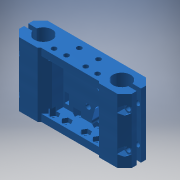
# Autodesk Inventor part: ChimeraXCarriageBushings
Saved by Autodesk Inventor 2016 (Build 200138000, 138)
## iProperties
Category: Print
Created: 2015-03-10
Part Number: ChimeraXCarriageBushings
Material: ABS Plastic
Document SubType Name: Modeling
Designer: Jack
Density: 1.06 g/cm^3
Appearance: Cyan
Mass: 40.4192 g
Surface Area: 204.208 cm^2
Volume: 38.1313 cm^3
Author: Jack
Title: Chimera X Carriage V6
Autodesk Inventor part; units mm, degrees
ref_plane "YZ Plane" through (0, 0, 0) normal (1, 0, 0) x (0, 1, 0)
ref_plane "XZ Plane" through (0, 0, 0) normal (0, 1, 0) x (-1, 0, 0)
sketch "Sketch1" plane through (0, 0, 0) normal (0, 0, 1) x (1, 0, 0)
  arc A0 (-6.0673, -1.5) -> (-6.0673, 1.5) centre (0, 0) ccw
  arc A1 (61.0673, 1.5) -> (61.0673, -1.5) centre (55, 0) ccw
  line L0 (-6.0673, -1.5) -> (-12, -1.5)
  line L1 (-12, -1.5) -> (-12, -10)
  line L2 (-12, -10) -> (11, -10)
  line L3 (11, -10) -> (11, 3)
  line L4 (11, 3) -> (44, 3)
  line L5 (44, 3) -> (44, -10)
  line L6 (44, -10) -> (67, -10)
  line L7 (67, -10) -> (67, -1.5)
  line L8 (67, -1.5) -> (61.0673, -1.5)
  line L9 (61.0673, 1.5) -> (67, 1.5)
  line L10 (67, 1.5) -> (67, 10)
  line L11 (67, 10) -> (44, 10)
  line L12 (44, 10) -> (44, 10)
  line L13 (44, 10) -> (11, 10)
  line L14 (11, 10) -> (11, 10)
  line L15 (11, 10) -> (-12, 10)
  line L16 (-12, 10) -> (-12, 1.5)
  line L17 (-12, 1.5) -> (-6.0673, 1.5)
  dimension "d0" = 12.5
  dimension "d1" = 55
  dimension "d2" = 1.5
  dimension "d4" = 10
  dimension "d5" = 11
  dimension "d6" = 10
  dimension "d8" = 13
  dimension "d9" = 7
  dimension "d147" = 12
  constraints: 36 end point, 12 perpendicular, 6 point on line, 4 equal length, 4 point on circle, 4 vertical alignment, 2 centre point, 2 horizontal alignment, 1 coincident, 1 equal radius, 1 horizontal, 1 parallel, 1 vertical
  measures "d0" diameter of A0
  measures "d1" distance of A1.centre point (0, 0)
  measures "d2" distance from line of point (0, 0) L0
  measures "d4" distance from line of L15 point (0, 0)
  measures "d5" distance from line of L14 point (0, 0)
  measures "d6" distance from line of L2 point (0, 0)
  measures "d8" distance of L2.end L3.end
  measures "d9" distance between parallel lines of L4 L13
  measures "d147" distance from line of point (0, 0) L16
extrude "Extrusion1" add sketch "Sketch1" along normal blind 45
chamfer "Chamfer1" distance 5 angle 45 6 edges at (-12, 10, 22.5) (-12, -10, 22.5) (67, -10, 22.5) (67, 10, 22.5) (44, -10, 22.5) (11, -10, 22.5)
sketch "Sketch2" plane through (-7, 10, 0) normal (0, 1, 0) x (1, 0, 0)
  line L0 (69, 0) -> (69, -45) projected
  line L1 (0, -45) -> (0, 0) projected
  line L2 (74, -45) -> (74, 0) projected
  line L3 (-5, 0) -> (-5, -45) projected
  line L4 (74, 0) -> (69, 0) projected
  line L5 (69, -45) -> (74, -45) projected
  point P0 (7, 0)
  point P1 (-2.5, -10)
  point P2 (-2.5, -35)
  point P3 (71.5, -10)
  point P4 (71.5, -35)
  dimension "d18" = 2.5
  dimension "d19" = 2.5
  dimension "d20" = 10
  dimension "d21" = 10
  constraints: 2 horizontal alignment, 2 vertical alignment
  measures "d18" distance from line of L1 point (-2.5, -10)
  measures "d19" distance from line of L0 point (71.5, -10)
  measures "d20" distance from line of L4 point (71.5, -10)
  measures "d21" distance from line of L5 point (71.5, -35)
hole "Hole1" at (-9.5, 10, 10) at (-9.5, 10, 35) at (64.5, 10, 10) at (64.5, 10, 35) direction (0, -1, 0) diameter 3.5 end through all counterbore diameter 7.3 counterbore depth 5
sketch "Sketch3" plane through (49, -10, 0) normal (0, -1, 0) x (1, 0, 0)
  circle A0 centre (15.5, 10) radius 1.75 projected
  circle A1 centre (15.5, 35) radius 1.75 projected
  circle A2 centre (-58.5, 35) radius 1.75 projected
  circle A3 centre (-58.5, 10) radius 1.75 projected
  line L0 (15.5, 13.1754) -> (18.25, 11.5877)
  line L1 (18.25, 11.5877) -> (18.25, 8.4123)
  line L2 (18.25, 8.4123) -> (15.5, 6.8246)
  line L3 (15.5, 6.8246) -> (12.75, 8.4123)
  line L4 (12.75, 8.4123) -> (12.75, 11.5877)
  line L5 (12.75, 11.5877) -> (15.5, 13.1754)
  line L6 (15.5, 31.8246) -> (12.75, 33.4123)
  line L7 (12.75, 33.4123) -> (12.75, 36.5877)
  line L8 (12.75, 36.5877) -> (15.5, 38.1754)
  line L9 (15.5, 38.1754) -> (18.25, 36.5877)
  line L10 (18.25, 36.5877) -> (18.25, 33.4123)
  line L11 (18.25, 33.4123) -> (15.5, 31.8246)
  circle A4 centre (-58.5, 10) radius 1.75 projected
  line L12 (-58.5, 6.8246) -> (-61.25, 8.4123)
  line L13 (-61.25, 8.4123) -> (-61.25, 11.5877)
  line L14 (-61.25, 11.5877) -> (-58.5, 13.1754)
  line L15 (-58.5, 13.1754) -> (-55.75, 11.5877)
  line L16 (-55.75, 11.5877) -> (-55.75, 8.4123)
  line L17 (-55.75, 8.4123) -> (-58.5, 6.8246)
  line L18 (-58.5, 38.1754) -> (-55.75, 36.5877)
  line L19 (-55.75, 36.5877) -> (-55.75, 33.4123)
  line L20 (-55.75, 33.4123) -> (-58.5, 31.8246)
  line L21 (-58.5, 31.8246) -> (-61.25, 33.4123)
  line L22 (-61.25, 33.4123) -> (-61.25, 36.5877)
  line L23 (-61.25, 36.5877) -> (-58.5, 38.1754)
  point P0 (-49, 0)
  point P1 (-58.5, 10)
  dimension "d29" = 5.5
  constraints: 48 end point, 4 coincident, 4 vertical, 3 parallel, 52 other
  measures "d29" distance between parallel lines of L4 L1
extrude "Extrusion2" cut sketch "Sketch3" against normal blind 5
sketch "Sketch5" plane through (-7, 10, 0) normal (0, 1, 0) x (1, 0, 0)
  line L0 (0, 0) -> (69, 0) projected
  line L1 (51, 0) -> (51, -45) projected
  point P0 (7, 0)
  point P1 (47.5, -22.5)
  point P2 (35.5, -31)
  point P3 (35.5, -14)
  dimension "d44" = 17
  dimension "d45" = 12
  dimension "d46" = 3.5
  dimension "d47" = 22.5
  dimension "d48" = 8.5
  constraints: 1 vertical alignment
  measures "d44" distance of point (35.5, -31) point (35.5, -14)
  measures "d45" horizontal distance of point (35.5, -14) point (47.5, -22.5)
  measures "d46" distance from line of L1 point (47.5, -22.5)
  measures "d47" distance from line of L0 point (47.5, -22.5)
  measures "d48" vertical distance of point (47.5, -22.5) point (35.5, -31)
hole "Hole3" at (40.5, 10, 22.5) at (28.5, 10, 31) at (28.5, 10, 14) direction (0, -1, 0) diameter 3.5 end through all counterbore diameter 7.3 counterbore depth 3.5
sketch "Sketch6" plane through (-7, 10, 0) normal (0, 1, 0) x (1, 0, 0)
  circle A0 centre (47.5, -22.5) radius 3.65 projected
  arc A1 (50.9105, -7.1631) -> (48.5, -4) centre (48.5, -6.5) ccw
  arc A2 (48.5, -41) -> (50.9105, -37.8369) centre (48.5, -38.5) ccw
  arc A3 (48.8388, -30.3064) -> (40.1612, -30.3064) centre (44.5, -31.5) ccw
  arc A4 (40.1612, -14.6936) -> (48.8388, -14.6936) centre (44.5, -13.5) ccw
  arc A5 (40.5, -4) -> (38.0895, -7.1631) centre (40.5, -6.5) ccw
  arc A6 (38.0895, -37.8369) -> (40.5, -41) centre (40.5, -38.5) ccw
  line L0 (40.5, -4) -> (48.5, -4)
  line L1 (50.9105, -7.1631) -> (48.8388, -14.6936)
  line L2 (38.0895, -7.1631) -> (40.1612, -14.6936)
  line L3 (48.8388, -30.3064) -> (50.9105, -37.8369)
  line L4 (40.1612, -30.3064) -> (38.0895, -37.8369)
  line L5 (40.5, -41) -> (48.5, -41)
  point P0 (7, 0)
  dimension "d136" = 9
  dimension "d138" = 4
  dimension "d139" = 9
  dimension "d140" = 9
  dimension "d141" = 18
  dimension "d142" = 3
  dimension "d143" = 7
  dimension "d144" = 7
  dimension "d145" = 5
  dimension "d146" = 4
  constraints: 12 end point, 12 point on circle, 12 tangent, 6 centre point, 3 equal radius, 3 vertical alignment, 2 horizontal alignment, 1 horizontal
  measures "d136" diameter of A3
  measures "d138" horizontal distance of A2.centre A3.centre
  measures "d139" vertical distance of A0.centre A3.centre
  measures "d140" diameter of A4
  measures "d141" distance of A3.centre A4.centre
  measures "d142" horizontal distance of A0.centre A4.centre
  measures "d143" vertical distance of A2.centre A3.centre
  measures "d144" vertical distance of A4.centre A1.centre
  measures "d145" diameter of A1
  measures "d146" horizontal distance of A4.centre A5.centre
extrude "Extrusion3" cut sketch "Sketch6" against normal up to surface (7 mm away) contours L1 A4 L2 A5 L0 A1 | L5 A6 L4 A3 L3 A2
sketch "Sketch7" plane through (0, 0, 45) normal (0, 0, 1) x (1, 0, 0)
  line L0 (11, -5) -> (6, -10) projected
  line L1 (11, -5) -> (11, 3) projected
  line L2 (11, 3) -> (44, 3) projected
  line L3 (44, 3) -> (44, -5) projected
  arc A0 (61.0673, 1.5) -> (61.0673, -1.5) centre (55, 0) ccw projected
  line L4 (7.3, -8.7) -> (47.7, -8.7)
  line L5 (44, -5) -> (49, -10) projected
  dimension "d66" = 8.7
  constraints: 2 end point, 2 point on line, 1 horizontal
  measures "d66" distance from line of A0.centre L4
extrude "Extrusion4" add sketch "Sketch7" against normal blind 5
sketch "Sketch8" plane through (0, 0, 0) normal (0, 0, -1) x (-1, 0, 0)
  line L0 (-11, -5) -> (-7.3, -8.7) projected
  line L1 (-11, 3) -> (-11, -5) projected
  line L2 (-31.5, 3) -> (-11, 3) projected
  line L3 (-44, -5) -> (-44, 3) projected
  line L4 (-47.7, -8.7) -> (-44, -5) projected
  line L5 (-47.7, -8.7) -> (-7.3, -8.7) projected
  line L6 (-31.5, 3) -> (-43.5, 3) projected
  line L7 (-44, 3) -> (-43.5, 3) projected
extrude "Extrusion5" add sketch "Sketch8" against normal blind 5
sketch "Sketch9" plane through (0, 0, 0) normal (0, 0, -1) x (-1, 0, 0)
  arc A0 (6.0673, 1.5) -> (6.0673, -1.5) centre (0, 0) ccw projected
  line L0 (12, 1.5) -> (12, 5) projected
  circle A1 centre (-34.25, 4.45) radius 1.75
  circle A2 centre (-34.25, -4.45) radius 1.75
  circle A3 centre (-20.75, 4.45) radius 1.75
  circle A4 centre (-20.75, -4.45) radius 1.75
  dimension "d71" = 3.5
  dimension "d72" = 13.5
  dimension "d73" = 8.9
  dimension "d74" = 4.45
  dimension "d76" = 32.75
  constraints: 4 centre point, 3 equal radius, 2 horizontal alignment, 2 vertical alignment
  measures "d71" diameter of A1
  measures "d72" distance of A3.centre A1.centre
  measures "d73" distance of A3.centre A4.centre
  measures "d74" vertical distance of A0.centre A3.centre
  measures "d76" distance from line of L0 A3.centre
extrude "Extrusion6" cut sketch "Sketch9" against normal up to surface (5 mm away)
sketch "Sketch10" plane through (0, 0, 45) normal (0, 0, 1) x (1, 0, 0)
  circle A0 centre (34.25, -4.45) radius 1.75 projected
  circle A1 centre (20.75, -4.45) radius 1.75 projected
  arc A2 (19.7702, 3) -> (21.7298, 3) centre (20.75, 4.45) ccw projected
  arc A3 (33.2702, 3) -> (35.2298, 3) centre (34.25, 4.45) ccw projected
  circle A4 centre (20.75, 4.45) radius 1.75 projected
  circle A5 centre (34.25, 4.45) radius 1.75 projected
extrude "Extrusion7" cut sketch "Sketch10" against normal up to surface (5 mm away)
sketch "Sketch11" plane through (0, 0, 40) normal (0, 0, -1) x (-1, 0, 0)
  arc A0 (-21.7298, 3) -> (-19.7702, 3) centre (-20.75, 4.45) ccw projected
  arc A1 (-35.2298, 3) -> (-33.2702, 3) centre (-34.25, 4.45) ccw projected
  circle A2 centre (-20.75, -4.45) radius 1.75 projected
  circle A3 centre (-34.25, -4.45) radius 1.75 projected
  line L0 (-31.5, 6.0377) -> (-31.5, 2.8623)
  line L1 (-31.5, 2.8623) -> (-34.25, 1.2746)
  line L2 (-34.25, 1.2746) -> (-37, 2.8623)
  line L3 (-37, 2.8623) -> (-37, 6.0377)
  line L4 (-37, 6.0377) -> (-34.25, 7.6254)
  line L5 (-34.25, 7.6254) -> (-31.5, 6.0377)
  line L6 (-31.0746, -4.45) -> (-32.6623, -7.2)
  line L7 (-32.6623, -7.2) -> (-35.8377, -7.2)
  line L8 (-35.8377, -7.2) -> (-37.4254, -4.45)
  line L9 (-37.4254, -4.45) -> (-35.8377, -1.7)
  line L10 (-35.8377, -1.7) -> (-32.6623, -1.7)
  line L11 (-32.6623, -1.7) -> (-31.0746, -4.45)
  line L12 (-23.9254, -4.45) -> (-22.3377, -1.7)
  line L13 (-22.3377, -1.7) -> (-19.1623, -1.7)
  line L14 (-19.1623, -1.7) -> (-17.5746, -4.45)
  line L15 (-17.5746, -4.45) -> (-19.1623, -7.2)
  line L16 (-19.1623, -7.2) -> (-22.3377, -7.2)
  line L17 (-22.3377, -7.2) -> (-23.9254, -4.45)
  line L18 (-23.5, 6.0377) -> (-20.75, 7.6254)
  line L19 (-20.75, 7.6254) -> (-18, 6.0377)
  line L20 (-18, 6.0377) -> (-18, 2.8623)
  line L21 (-18, 2.8623) -> (-20.75, 1.2746)
  line L22 (-20.75, 1.2746) -> (-23.5, 2.8623)
  line L23 (-23.5, 2.8623) -> (-23.5, 6.0377)
  point P0 (0, 0)
  dimension "d81" = 5.5
  constraints: 48 end point, 4 coincident, 3 equal length, 2 horizontal, 2 vertical, 52 other
  measures "d81" distance between parallel lines of L8 L11
extrude "Extrusion8" cut sketch "Sketch11" along normal blind 3.5 and the other way blind 3
sketch "Sketch12" plane through (0, 0, 5) normal (0, 0, 1) x (1, 0, 0)
  circle A0 centre (34.25, 4.45) radius 1.75 projected
  line L0 (31.5, 6.0377) -> (31.5, 2.8623) projected
  line L1 (34.25, 7.6254) -> (31.5, 6.0377) projected
  line L2 (37, 6.0377) -> (34.25, 7.6254) projected
  line L3 (37, 2.8623) -> (37, 6.0377) projected
  line L4 (34.25, 1.2746) -> (37, 2.8623) projected
  line L5 (31.5, 2.8623) -> (34.25, 1.2746) projected
  circle A1 centre (34.25, -4.45) radius 1.75 projected
  line L6 (31.0746, -4.45) -> (32.6623, -7.2) projected
  line L7 (32.6623, -1.7) -> (31.0746, -4.45) projected
  line L8 (35.8377, -1.7) -> (32.6623, -1.7) projected
  line L9 (37.4254, -4.45) -> (35.8377, -1.7) projected
  line L10 (35.8377, -7.2) -> (37.4254, -4.45) projected
  line L11 (32.6623, -7.2) -> (35.8377, -7.2) projected
  circle A2 centre (20.75, 4.45) radius 1.75 projected
  line L12 (23.5, 6.0377) -> (20.75, 7.6254) projected
  line L13 (23.5, 2.8623) -> (23.5, 6.0377) projected
  line L14 (20.75, 1.2746) -> (23.5, 2.8623) projected
  line L15 (18, 2.8623) -> (20.75, 1.2746) projected
  line L16 (18, 6.0377) -> (18, 2.8623) projected
  line L17 (20.75, 7.6254) -> (18, 6.0377) projected
  circle A3 centre (20.75, -4.45) radius 1.75 projected
  line L18 (23.9254, -4.45) -> (22.3377, -1.7) projected
  line L19 (22.3377, -7.2) -> (23.9254, -4.45) projected
  line L20 (19.1623, -7.2) -> (22.3377, -7.2) projected
  line L21 (17.5746, -4.45) -> (19.1623, -7.2) projected
  line L22 (19.1623, -1.7) -> (17.5746, -4.45) projected
  line L23 (22.3377, -1.7) -> (19.1623, -1.7) projected
  point P0 (0, 0)
extrude "Extrusion9" cut sketch "Sketch12" along normal blind 3.5 and the other way blind 3 contours A0 | L1 L2 L3 L4 L5 L0 | A1 | L7 L8 L9 L10 L11 L6 | A2 | L13 L14 L15 L16 L17 L12 | A3 | L19 L20 L21 L22 L23 L18
ref_plane "Work Plane1" through (0, 0, 2) normal (0, 0, -1) x (-1, 0, 0)
sketch "Sketch15" plane through (0, 0, 2) normal (0, 0, -1) x (-1, 0, 0)
  circle A0 centre (-20.75, 4.45) radius 1.75 projected
  circle A1 centre (-20.75, -4.45) radius 1.75 projected
  circle A2 centre (-34.25, -4.45) radius 1.75 projected
  circle A3 centre (-34.25, 4.45) radius 1.75 projected
  line L0 (-6, -10) -> (-7.3, -8.7) projected
  line L1 (-6, -10) -> (7, -10) projected
  line L2 (12, -5) -> (7, -10) projected
  line L3 (12, -5) -> (12, -1.5) projected
  line L4 (12, -1.5) -> (6.0673, -1.5) projected
  arc A4 (6.0673, 1.5) -> (6.0673, -1.5) centre (0, 0) ccw projected
  line L5 (6.0673, 1.5) -> (12, 1.5) projected
  line L6 (12, 1.5) -> (12, 5) projected
  line L7 (7, 10) -> (12, 5) projected
  line L8 (7, 10) -> (-62, 10) projected
  line L9 (-67, 5) -> (-62, 10) projected
  line L10 (-67, 5) -> (-67, 1.5) projected
  line L11 (-67, 1.5) -> (-61.0673, 1.5) projected
  arc A5 (-61.0673, -1.5) -> (-61.0673, 1.5) centre (-55, 0) ccw projected
  line L12 (-61.0673, -1.5) -> (-67, -1.5) projected
  line L13 (-67, -1.5) -> (-67, -5) projected
  line L14 (-62, -10) -> (-67, -5) projected
  line L15 (-62, -10) -> (-49, -10) projected
  line L16 (-47.7, -8.7) -> (-49, -10) projected
  line L17 (-47.7, -8.7) -> (-7.3, -8.7) projected
  line L18 (7, 10) -> (-62, 10) projected
  line L19 (-40, 10) -> (-40, 20.5)
  line L20 (-40, 20.5) -> (-14, 20.5)
  line L21 (-14, 20.5) -> (-14, 10)
  circle A6 centre (-37, 15) radius 1.75
  circle A7 centre (-18, 15) radius 1.75
  dimension "d103" = 26
  dimension "d104" = 26
  dimension "d105" = 10.5
  dimension "d106" = 3.5
  dimension "d107" = 19
  dimension "d108" = 5.5
  dimension "d109" = 3
  constraints: 6 end point, 3 perpendicular, 2 centre point, 2 point on line, 1 equal radius, 1 horizontal alignment
  measures "d103" distance between parallel lines of L6 L21
  measures "d104" distance of L19.end L20.end
  measures "d105" distance between parallel lines of L8 L20
  measures "d106" diameter of A6
  measures "d107" distance of A7.centre A6.centre
  measures "d108" distance from line of L20 A7.centre
  measures "d109" distance from line of L19 A6.centre
extrude "Extrusion12" add sketch "Sketch15" against normal blind 5 contours L8 L19 L20 L21
chamfer "Chamfer3" distance 2.5 angle 45 1 edges at (35.5253, 10, 7)
sketch "Sketch16" plane through (0, 0, 7) normal (0, 0, 1) x (1, 0, 0)
  circle A0 centre (18, 15) radius 1.75 projected
  circle A1 centre (37, 15) radius 1.75 projected
  line L0 (18, 11.8246) -> (15.25, 13.4123)
  line L1 (15.25, 13.4123) -> (15.25, 16.5877)
  line L2 (15.25, 16.5877) -> (18, 18.1754)
  line L3 (18, 18.1754) -> (20.75, 16.5877)
  line L4 (20.75, 16.5877) -> (20.75, 13.4123)
  line L5 (20.75, 13.4123) -> (18, 11.8246)
  line L6 (37, 11.8246) -> (34.25, 13.4123)
  line L7 (34.25, 13.4123) -> (34.25, 16.5877)
  line L8 (34.25, 16.5877) -> (37, 18.1754)
  line L9 (37, 18.1754) -> (39.75, 16.5877)
  line L10 (39.75, 16.5877) -> (39.75, 13.4123)
  line L11 (39.75, 13.4123) -> (37, 11.8246)
  point P0 (0, 0)
  dimension "d115" = 5.5
  constraints: 24 end point, 2 coincident, 1 horizontal alignment, 1 parallel, 1 vertical, 26 other
  measures "d115" distance between parallel lines of L10 L7
extrude "Extrusion13" cut sketch "Sketch16" against normal blind 3
sketch "Sketch17" plane through (0, 0, 45) normal (0, 0, 1) x (1, 0, 0)
  line L0 (67, -5) -> (67, -1.5) projected
  line L1 (7.3, -8.7) -> (47.7, -8.7) projected
  circle A0 centre (12.25, -4.7) radius 1.75
  circle A1 centre (42.75, -4.7) radius 1.75
  dimension "d118" = 3.5
  dimension "d121" = 4
  dimension "d148" = 30.5
  dimension "d149" = 24.25
  constraints: 2 centre point, 1 equal radius, 1 horizontal alignment
  measures "d118" diameter of A0
  measures "d121" distance from line of L1 A1.centre
  measures "d148" distance of A1.centre A0.centre
  measures "d149" distance from line of L0 A1.centre
extrude "Extrusion14" cut sketch "Sketch17" against normal up to surface (5 mm away)
sketch "Sketch18" plane through (0, 0, 0) normal (0, 0, -1) x (-1, 0, 0)
  arc A0 (-44.3676, -5.3676) -> (-44, -3.4753) centre (-42.75, -4.7) ccw projected
  circle A1 centre (-42.75, -4.7) radius 1.75 projected
  arc A2 (-11, -3.4753) -> (-10.6324, -5.3676) centre (-12.25, -4.7) ccw projected
  circle A3 centre (-12.25, -4.7) radius 1.75 projected
  arc A4 (-10.6324, -5.3676) -> (-11, -3.4753) centre (-12.25, -4.7) ccw projected
  arc A5 (-44, -3.4753) -> (-44.3676, -5.3676) centre (-42.75, -4.7) ccw projected
extrude "Extrusion15" cut sketch "Sketch18" against normal up to surface (5 mm away)
sketch "Sketch19" plane through (0, 0, 5) normal (0, 0, 1) x (1, 0, 0)
  circle A0 centre (42.75, -4.7) radius 1.75 projected
  circle A1 centre (12.25, -4.7) radius 1.75 projected
  line L0 (15.4254, -4.7) -> (13.8377, -7.45)
  line L1 (13.8377, -7.45) -> (10.6623, -7.45)
  line L2 (10.6623, -7.45) -> (9.0746, -4.7)
  line L3 (9.0746, -4.7) -> (10.6623, -1.95)
  line L4 (10.6623, -1.95) -> (13.8377, -1.95)
  line L5 (13.8377, -1.95) -> (15.4254, -4.7)
  line L6 (39.5746, -4.7) -> (41.1623, -1.95)
  line L7 (41.1623, -1.95) -> (44.3377, -1.95)
  line L8 (44.3377, -1.95) -> (45.9254, -4.7)
  line L9 (45.9254, -4.7) -> (44.3377, -7.45)
  line L10 (44.3377, -7.45) -> (41.1623, -7.45)
  line L11 (41.1623, -7.45) -> (39.5746, -4.7)
  point P0 (44, -5.9247)
  point P1 (44, -3.4753)
  point P2 (11, -3.4753)
  point P3 (11, -5.9247)
  point P4 (0, 0)
  dimension "d126" = 5.5
  constraints: 24 end point, 2 coincident, 2 horizontal, 1 collinear, 26 other
  measures "d126" distance between parallel lines of L1 L4
extrude "Extrusion16" cut sketch "Sketch19" against normal blind 3 and the other way blind 3 contours A0 | A1 | L0 L1 L2 L3 L4 L5 | L6 L7 L8 L9 L10 L11
sketch "Sketch20" plane through (0, 0, 40) normal (0, 0, -1) x (-1, 0, 0)
  circle A0 centre (-12.25, -4.7) radius 1.75 projected
  line L0 (-15.4254, -4.7) -> (-13.8377, -7.45) projected
  line L1 (-13.8377, -1.95) -> (-15.4254, -4.7) projected
  line L2 (-10.6623, -1.95) -> (-13.8377, -1.95) projected
  line L3 (-9.0746, -4.7) -> (-10.6623, -1.95) projected
  line L4 (-10.6623, -7.45) -> (-9.0746, -4.7) projected
  line L5 (-13.8377, -7.45) -> (-10.6623, -7.45) projected
  circle A1 centre (-42.75, -4.7) radius 1.75 projected
  line L6 (-39.5746, -4.7) -> (-41.1623, -1.95) projected
  line L7 (-41.1623, -7.45) -> (-39.5746, -4.7) projected
  line L8 (-44.3377, -7.45) -> (-41.1623, -7.45) projected
  line L9 (-45.9254, -4.7) -> (-44.3377, -7.45) projected
  line L10 (-44.3377, -1.95) -> (-45.9254, -4.7) projected
  line L11 (-41.1623, -1.95) -> (-44.3377, -1.95) projected
  point P0 (0, 0)
extrude "Extrusion17" cut sketch "Sketch20" along normal blind 3 and the other way blind 3 contours A0 | L1 L2 L3 L4 L5 L0 | A1 | L7 L8 L9 L10 L11 L6
sketch "Sketch21" plane through (37.5, 3, 13.5) normal (0, -1, 0) x (1, 0, 0)
  line L0 (-22.5, 1.5) -> (-25.5, 1.5)
  line L1 (-25.5, 1.5) -> (-25.5, -5.5)
  line L2 (-25.5, -5.5) -> (-22.5, -5.5)
  line L3 (-22.5, -5.5) -> (-22.5, 1.5)
  line L4 (-26.5, -5.5) -> (-26.5, 23.5) projected
  line L5 (-30.2, -8.5) -> (10.2, -8.5) projected
  point P0 (-37.5, -13.5)
  dimension "d150" = 3
  dimension "d151" = 7
  dimension "d152" = 1
  dimension "d153" = 3
  constraints: 8 end point, 2 parallel, 1 horizontal, 1 perpendicular
  measures "d150" distance of L2.end L1.end
  measures "d151" distance of L1.end L0.end
  measures "d152" distance between parallel lines of L4 L1
  measures "d153" distance between parallel lines of L5 L2
extrude "Extrusion18" cut sketch "Sketch21" against normal up to surface (7 mm away)
body "Solid1"
